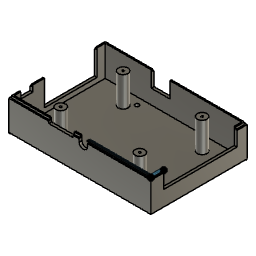
CaseTop (Autodesk Fusion 360 design; units mm, degrees)
Autodesk Fusion 360 part; units mm, degrees
sketch "Sketch1" plane through (0, 0, 0) normal (0, 0, 1) x (1, 0, 0)
  line L0 (0, 0) -> (102.5, 0)
  line L1 (102.5, 0) -> (102.5, 69.5)
  line L2 (102.5, 69.5) -> (0, 69.5)
  line L3 (0, 69.5) -> (0, 0)
  dimension "d1" = 69.5
  dimension "d2" = 102.5
  constraint horizontal L0
  constraint vertical L1
  constraint horizontal L2
  constraint vertical L3
  constraint coincident L0.start L3.end
  measures "d1" distance of L0 L2
  measures "d2" distance of L1 L3
extrude "Extrude1" add sketch "Sketch1" along normal blind 24
shell "Shell1" thickness 2 removed faces 1 at (34.1667, 46.3333, 24)
sketch "Sketch2" plane through (0, 0, 2) normal (0, 0, 1) x (-1, 0, 0)
  line L0 (-2, -67.5) -> (-2, -2)
  line L1 (-2, -2) -> (-100.5, -2)
  line L2 (-100.5, -2) -> (-100.5, -67.5)
  line L3 (-100.5, -67.5) -> (-2, -67.5)
  circle A0 centre (-82.25, -57.25) radius 3.5
  dimension "d6" = 7
  dimension "d7" = 18.25
  dimension "d8" = 10.25
  measures "d6" diameter of A0
  measures "d7" distance of L2 A0.centre
  measures "d8" distance of L3 A0.centre
extrude "Extrude2" add sketch "Sketch2" along normal blind 21.5 contours A0
sketch "Sketch5" plane through (0, 0, 23.5) normal (0, 0, 1) x (-1, 0, 0)
  circle A0 centre (-82.25, -57.25) radius 3.5
  circle A1 centre (-82.25, -57.25) radius 0.75
  dimension "d16" = 1.5
  constraint concentric A0 A1
  measures "d16" diameter of A1
extrude "Extrude4" cut sketch "Sketch5" against normal blind 8 contours A1
pattern_linear "R-Pattern1" count 2 spacing 57 along (-1, 0, 0) count 2 spacing 45 along (0, -1, 0) of "Extrude2", "Extrude4"
sketch "Sketch21" plane through (2, 0, 0) normal (1, 0, 0) x (0, 1, 0)
  line L0 (2, 2) -> (67.5, 2)
  line L1 (67.5, 2) -> (67.5, 24)
  line L2 (67.5, 24) -> (2, 24)
  line L3 (2, 24) -> (2, 2)
  line L4 (23.75, 24) -> (61.75, 24)
  line L5 (61.75, 24) -> (61.75, 5.5)
  line L6 (61.75, 5.5) -> (23.75, 5.5)
  line L7 (23.75, 5.5) -> (23.75, 24)
  dimension "d70" = 18.5
  dimension "d71" = 5.75
  dimension "d72" = 21.75
  constraint horizontal L4
  constraint vertical L5
  constraint horizontal L6
  constraint vertical L7
  constraint coincident L2 L4.start
  measures "d70" distance of L4 L6
  measures "d71" distance of L1 L5
  measures "d72" distance of L3 L7
extrude "Extrude17" cut sketch "Sketch21" against normal blind 2 contours L2 L4 L5 L6 L7
sketch "Sketch22" plane through (2, 0, 0) normal (1, 0, 0) x (0, 1, 0)
  line L0 (23.75, 5.5) -> (23.75, 24)
  line L1 (23.75, 24) -> (2, 24)
  line L2 (2, 24) -> (2, 2)
  line L3 (2, 2) -> (67.5, 2)
  line L4 (67.5, 2) -> (67.5, 24)
  line L5 (67.5, 24) -> (61.75, 24)
  line L6 (61.75, 24) -> (61.75, 5.5)
  line L7 (61.75, 5.5) -> (23.75, 5.5)
  line L8 (6.75, 24) -> (15.25, 24)
  line L9 (15.25, 24) -> (15.25, 19.5)
  line L10 (15.25, 19.5) -> (6.75, 19.5)
  line L11 (6.75, 19.5) -> (6.75, 24)
  dimension "d75" = 4.5
  dimension "d76" = 4.75
  dimension "d77" = 8.5
  constraint horizontal L8
  constraint vertical L9
  constraint horizontal L10
  constraint vertical L11
  constraint coincident L1 L8.start
  measures "d75" distance of L8 L10
  measures "d76" distance of L2 L11
  measures "d77" distance of L9 L11
extrude "Extrude18" cut sketch "Sketch22" against normal blind 2 contours L1 L8 L9 L10 L11
sketch "Sketch23" plane through (0, 67.5, 0) normal (0, -1, 0) x (1, 0, 0)
  line L0 (2, 2) -> (100.5, 2)
  line L1 (100.5, 2) -> (100.5, 24)
  line L2 (100.5, 24) -> (2, 24)
  line L3 (2, 24) -> (2, 2)
  line L4 (35.25, 24) -> (48.75, 24)
  line L5 (48.75, 24) -> (48.75, 12.5)
  line L6 (48.75, 12.5) -> (35.25, 12.5)
  line L7 (35.25, 12.5) -> (35.25, 24)
  dimension "d80" = 33.25
  dimension "d81" = 13.5
  dimension "d82" = 11.5
  constraint horizontal L4
  constraint vertical L5
  constraint horizontal L6
  constraint vertical L7
  constraint coincident L2 L4.start
  measures "d80" distance of L3 L7
  measures "d81" distance of L5 L7
  measures "d82" distance of L4 L6
extrude "Extrude19" cut sketch "Sketch23" against normal blind 2 contours L2 L4 L5 L6 L7
sketch "Sketch24" plane through (102.5, 0, 0) normal (1, 0, 0) x (0, 1, 0)
  line L0 (0, 0) -> (69.5, 0)
  line L1 (69.5, 0) -> (69.5, 24)
  line L2 (69.5, 24) -> (0, 24)
  line L3 (0, 24) -> (0, 0)
  line L4 (62.25, 24) -> (9.25, 24)
  line L5 (9.25, 24) -> (9.25, 12)
  line L6 (9.25, 12) -> (62.25, 12)
  line L7 (62.25, 12) -> (62.25, 24)
  dimension "d85" = 7.25
  dimension "d86" = 9.25
  dimension "d87" = 12
  constraint horizontal L4
  constraint vertical L5
  constraint horizontal L6
  constraint vertical L7
  constraint coincident L2 L4.start
  measures "d85" distance of L1 L7
  measures "d86" distance of L3 L5
  measures "d87" distance of L4 L6
extrude "Extrude20" cut sketch "Sketch24" against normal blind 2 contours L2 L4 L5 L6 L7
sketch "Sketch25" plane through (0, 0, 0) normal (0, -1, 0) x (1, 0, 0)
  line L0 (0, 0) -> (102.5, 0)
  line L1 (102.5, 0) -> (102.5, 24)
  line L2 (102.5, 24) -> (0, 24)
  line L3 (0, 24) -> (0, 0)
  line L4 (46.25, 21) -> (28.75, 21)
  line L5 (28.75, 21) -> (28.75, 24)
  line L6 (28.75, 24) -> (46.25, 24)
  line L7 (46.25, 24) -> (46.25, 21)
  dimension "d90" = 3
  dimension "d91" = 28.75
  dimension "d92" = 17.5
  constraint horizontal L4
  constraint vertical L5
  constraint horizontal L6
  constraint vertical L7
  constraint coincident L2 L5.end
  measures "d90" distance of L4 L6
  measures "d91" distance of L3 L5
  measures "d92" distance of L5 L7
extrude "Extrude21" cut sketch "Sketch25" against normal blind 2 contours L2 L4 L5 L6 L7
sketch "Sketch26" plane through (0, 0, 0) normal (0, -1, 0) x (1, 0, 0)
  line L0 (28.75, 21) -> (28.75, 24)
  line L1 (28.75, 24) -> (0, 24)
  line L2 (0, 24) -> (0, 0)
  line L3 (0, 0) -> (102.5, 0)
  line L4 (102.5, 0) -> (102.5, 24)
  line L5 (102.5, 24) -> (46.25, 24)
  line L6 (46.25, 24) -> (46.25, 21)
  line L7 (46.25, 21) -> (28.75, 21)
  line L8 (56.75, 20.35) -> (50.75, 20.35)
  line L9 (50.75, 20.35) -> (50.75, 24)
  line L10 (50.75, 24) -> (56.75, 24)
  line L11 (56.75, 24) -> (56.75, 20.35)
  circle A0 centre (53.75, 20.35) radius 3
  dimension "d95" = 50.75
  dimension "d96" = 45.75
  dimension "d97" = 3.65
  constraint horizontal L8
  constraint vertical L9
  constraint horizontal L10
  constraint vertical L11
  constraint coincident L5 L9.end
  constraint coincident L8.end A0
  constraint tangent L9 A0
  constraint coincident L8.start A0
  measures "d95" distance of L2 L9
  measures "d96" distance of L4 L11
  measures "d97" distance of L8 L10
extrude "Extrude22" cut sketch "Sketch26" against normal blind 2 contours L5 L9 L10 L11 A0 | L8 A0 | L8 A0
sketch "Sketch32" plane through (0, 0, 24) normal (0, 0, 1) x (-1, 0, 0)
  line L0 (-56.75, -2) -> (-56.75, 0)
  line L1 (-56.75, 0) -> (-102.5, 0)
  line L2 (-102.5, 0) -> (-102.5, -9.25)
  line L3 (-102.5, -9.25) -> (-100.5, -9.25)
  line L4 (-100.5, -9.25) -> (-100.5, -2)
  line L5 (-100.5, -2) -> (-56.75, -2)
  line L6 (-102.5, 0) -> (-56.75, 0)
  line L7 (-56.75, 0) -> (-56.75, -1)
  line L8 (-56.75, -1) -> (-102.5, -1)
  line L9 (-102.5, -1) -> (-102.5, 0)
  line L10 (-102.5, -9.25) -> (-101.5, -9.25)
  line L11 (-101.5, -9.25) -> (-101.5, 0)
  line L12 (-101.5, 0) -> (-102.5, 0)
  line L13 (-102.5, 0) -> (-102.5, -9.25)
  constraint horizontal L6
  constraint vertical L7
  constraint horizontal L8
  constraint vertical L9
  constraint midpoint L0 L7.end
  constraint coincident L1.end L2.start
  constraint horizontal L10
  constraint vertical L11
  constraint horizontal L12
  constraint vertical L13
  constraint coincident L6 L11.end
  constraint coincident L2.end L3.start
extrude "Extrude26" cut sketch "Sketch32" against normal blind 1.6 contours L0 L1 L6 L7 L8 L11 | L2 L3 L8 L10 L11 L13 | L1 L2 L6 L8 L9 L11 L12 L13
sketch "Sketch34" plane through (0, 0, 24) normal (0, 0, 1) x (-1, 0, 0)
  line L0 (-50.75, 0) -> (-50.75, -2)
  line L1 (-50.75, -2) -> (-46.25, -2)
  line L2 (-46.25, -2) -> (-46.25, 0)
  line L3 (-46.25, 0) -> (-50.75, 0)
  line L4 (-50.75, 0) -> (-46.25, 0)
  line L5 (-46.25, 0) -> (-46.25, -1)
  line L6 (-46.25, -1) -> (-50.75, -1)
  line L7 (-50.75, -1) -> (-50.75, 0)
  constraint horizontal L4
  constraint vertical L5
  constraint horizontal L6
  constraint vertical L7
  constraint midpoint L2 L5.end
  constraint coincident L0.start L3.end
extrude "Extrude27" cut sketch "Sketch34" against normal blind 1.6 contours L0 L2 L3 L4 L5 L6 L7
sketch "Sketch35" plane through (0, 0, 24) normal (0, 0, 1) x (-1, 0, 0)
  line L0 (-28.75, 0) -> (-28.75, -2)
  line L1 (-28.75, -2) -> (-2, -2)
  line L2 (-2, -2) -> (-2, -6.75)
  line L3 (-2, -6.75) -> (0, -6.75)
  line L4 (0, -6.75) -> (0, 0)
  line L5 (0, 0) -> (-28.75, 0)
  line L6 (-28.75, 0) -> (0, 0)
  line L7 (0, 0) -> (0, -1)
  line L8 (0, -1) -> (-28.75, -1)
  line L9 (-28.75, -1) -> (-28.75, 0)
  line L10 (0, -6.75) -> (-1, -6.75)
  line L11 (-1, -6.75) -> (-1, 0)
  line L12 (-1, 0) -> (0, 0)
  line L13 (0, 0) -> (0, -6.75)
  constraint horizontal L6
  constraint vertical L7
  constraint horizontal L8
  constraint vertical L9
  constraint coincident L4 L7.end
  constraint coincident L0.start L5.end
  constraint horizontal L10
  constraint vertical L11
  constraint horizontal L12
  constraint vertical L13
  constraint coincident L5 L11.end
  constraint coincident L3.end L4.start
extrude "Extrude28" cut sketch "Sketch35" against normal blind 1.6 contours L0 L5 L6 L8 L9 L11 | L4 L5 L6 L7 L8 L11 L12 L13 | L3 L4 L8 L10 L11 L13
sketch "Sketch36" plane through (0, 0, 24) normal (0, 0, 1) x (-1, 0, 0)
  line L0 (0, -15.25) -> (-2, -15.25)
  line L1 (-2, -15.25) -> (-2, -23.75)
  line L2 (-2, -23.75) -> (0, -23.75)
  line L3 (0, -23.75) -> (0, -15.25)
  line L4 (-1, -15.25) -> (0, -15.25)
  line L5 (0, -15.25) -> (0, -23.75)
  line L6 (0, -23.75) -> (-1, -23.75)
  line L7 (-1, -23.75) -> (-1, -15.25)
  constraint horizontal L4
  constraint vertical L5
  constraint horizontal L6
  constraint vertical L7
  constraint coincident L2.end L3.start
  constraint midpoint L0 L4.start
extrude "Extrude29" cut sketch "Sketch36" against normal blind 1.6 contours L0 L2 L3 L4 L5 L6 L7
sketch "Sketch37" plane through (0, 0, 24) normal (0, 0, 1) x (-1, 0, 0)
  line L0 (-35.25, -67.5) -> (-35.25, -69.5)
  line L1 (-35.25, -69.5) -> (0, -69.5)
  line L2 (0, -69.5) -> (0, -61.75)
  line L3 (0, -61.75) -> (-2, -61.75)
  line L4 (-2, -61.75) -> (-2, -67.5)
  line L5 (-2, -67.5) -> (-35.25, -67.5)
  line L6 (-35.25, -68.5) -> (0, -68.5)
  line L7 (0, -68.5) -> (0, -69.5)
  line L8 (0, -69.5) -> (-35.25, -69.5)
  line L9 (-35.25, -69.5) -> (-35.25, -68.5)
  line L10 (0, -61.75) -> (-1, -61.75)
  line L11 (-1, -61.75) -> (-1, -69.5)
  line L12 (-1, -69.5) -> (0, -69.5)
  line L13 (0, -69.5) -> (0, -61.75)
  constraint horizontal L6
  constraint vertical L7
  constraint horizontal L8
  constraint vertical L9
  constraint coincident L1.end L2.start
  constraint midpoint L0 L6.start
  constraint horizontal L10
  constraint vertical L11
  constraint horizontal L12
  constraint vertical L13
  constraint coincident L8 L11.end
  constraint coincident L2.end L3.start
extrude "Extrude30" cut sketch "Sketch37" against normal blind 1.6 contours L0 L1 L6 L8 L9 L11 | L2 L3 L6 L10 L11 L13 | L1 L2 L6 L7 L8 L11 L12 L13
sketch "Sketch38" plane through (0, 0, 24) normal (0, 0, 1) x (-1, 0, 0)
  line L0 (-100.5, -62.25) -> (-102.5, -62.25)
  line L1 (-102.5, -62.25) -> (-102.5, -69.5)
  line L2 (-102.5, -69.5) -> (-48.75, -69.5)
  line L3 (-48.75, -69.5) -> (-48.75, -67.5)
  line L4 (-48.75, -67.5) -> (-100.5, -67.5)
  line L5 (-100.5, -67.5) -> (-100.5, -62.25)
  line L6 (-102.5, -69.5) -> (-101.5, -69.5)
  line L7 (-101.5, -69.5) -> (-101.5, -62.25)
  line L8 (-101.5, -62.25) -> (-102.5, -62.25)
  line L9 (-102.5, -62.25) -> (-102.5, -69.5)
  line L10 (-48.75, -68.5) -> (-102.5, -68.5)
  line L11 (-102.5, -68.5) -> (-102.5, -69.5)
  line L12 (-102.5, -69.5) -> (-48.75, -69.5)
  line L13 (-48.75, -69.5) -> (-48.75, -68.5)
  constraint horizontal L6
  constraint vertical L7
  constraint horizontal L8
  constraint vertical L9
  constraint midpoint L0 L7.end
  constraint coincident L1.end L2.start
  constraint horizontal L10
  constraint vertical L11
  constraint horizontal L12
  constraint vertical L13
  constraint midpoint L3 L10.start
extrude "Extrude31" cut sketch "Sketch38" against normal blind 1.6 contours L0 L1 L7 L8 L9 L10 | L2 L3 L7 L10 L12 L13 | L1 L2 L6 L7 L9 L10 L11 L12
sketch "Sketch40" plane through (0, 0, 0) normal (0, 0, -1) x (1, 0, 0)
  line L0 (0, 0) -> (0, -69.5)
  line L1 (0, -69.5) -> (102.5, -69.5)
  line L2 (102.5, -69.5) -> (102.5, 0)
  line L3 (102.5, 0) -> (0, 0)
  circle A0 centre (30.25, -62.35) radius 1.45
  dimension "d122" = 2.9
  dimension "d123" = 7.15
  dimension "d124" = 30.25
  measures "d122" diameter of A0
  measures "d123" distance of L1 A0.centre
  measures "d124" distance of L0 A0.centre
extrude "Extrude32" cut sketch "Sketch40" against normal blind 2 contours A0
fillet "Fillet2" radius 1 4 edges at (51.25, 0, 0) (0, 34.75, 0) (51.25, 69.5, 0) (102.5, 34.75, 0)
equation "d1 = 65 mm + 4.5 mm"
equation "d2 = 98 mm + 4.5 mm"
equation "d3 = 22 mm + 2 mm"
equation "d85 = 5 mm + 2.25 mm"
equation "d86 = 7 mm + 2.25 mm"
equation "d95 = 48.5 mm + 2.25 mm"
equation "d96 = 43.5 mm + 2.25 mm"
equation "d97 = 5.25 mm - 1.6 mm"
equation "d123 = 4.9 mm + 2.25 mm"
equation "d124 = 28 mm + 2.25 mm"
